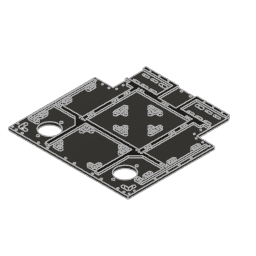
SumoBot-Chassis_5mm (Autodesk Fusion 360 design; units mm, degrees)
part number: 2026-04-02-11-57-34-569
Autodesk Fusion 360 part; units mm, degrees
(part 1 of 2)
sketch "Sketch1" plane through (0, 0, 0) normal (0, 0, 1) x (1, 0, 0)
  line L0 (67.5, 102.5) -> (-72.5, 102.5)
  line L1 (-102.5, 47.5) -> (-102.5, -97.5)
  line L2 (-102.5, -97.5) -> (97.5, -97.5)
  line L3 (97.5, -97.5) -> (97.5, 47.5)
  line L4 (-72.5, 102.5) -> (-72.5, 52.5)
  line L5 (67.5, 102.5) -> (67.5, 52.5)
  line L6 (-65.9, 77.5526) -> (-58.475, 77.6068)
  line L7 (-65.9, 74.3526) -> (-58.4517, 74.4069)
  line L8 (-51.9, 77.5526) -> (-44.1, 77.5526)
  line L9 (-51.9, 74.3526) -> (-44.1, 74.3526)
  arc A0 (-65.9, 77.5526) -> (-65.9, 74.3526) centre (-65.9, 75.9526) ccw
  arc A1 (-58.4517, 74.4069) -> (-58.475, 77.6068) centre (-58.4634, 76.0069) ccw
  arc A2 (-51.9, 77.5526) -> (-51.9, 74.3526) centre (-51.9, 75.9526) ccw
  arc A3 (-44.1, 74.3526) -> (-44.1, 77.5526) centre (-44.1, 75.9526) ccw
  arc A4 (-44.1, 90.4) -> (-44.1, 93.6) centre (-44.1, 92) ccw
  line L10 (-51.9, 90.4) -> (-44.1, 90.4)
  line L11 (-51.9, 93.6) -> (-44.1, 93.6)
  arc A5 (-51.9, 93.6) -> (-51.9, 90.4) centre (-51.9, 92) ccw
  line L12 (-65.9, 93.6) -> (-58.1, 93.6)
  arc A6 (-58.1, 90.4) -> (-58.1, 93.6) centre (-58.1, 92) ccw
  line L13 (-65.9, 90.4) -> (-58.1, 90.4)
  arc A7 (-65.9, 93.6) -> (-65.9, 90.4) centre (-65.9, 92) ccw
  line L14 (39.1, 74.3526) -> (46.9, 74.3526)
  arc A8 (39.1, 77.5526) -> (39.1, 74.3526) centre (39.1, 75.9526) ccw
  line L15 (39.1, 77.5526) -> (46.9, 77.5526)
  arc A9 (46.9, 74.3526) -> (46.9, 77.5526) centre (46.9, 75.9526) ccw
  arc A10 (53.1, 77.6) -> (53.1, 74.4) centre (53.1, 76) ccw
  line L16 (53.1, 74.4) -> (60.9, 74.4)
  line L17 (53.1, 77.6) -> (60.9, 77.6)
  arc A11 (60.9, 74.4) -> (60.9, 77.6) centre (60.9, 76) ccw
  arc A12 (39.1, 93.6474) -> (39.1, 90.4474) centre (39.1, 92.0474) ccw
  line L18 (39.1, 90.4474) -> (46.9, 90.4474)
  line L19 (39.1, 93.6474) -> (46.9, 93.6474)
  arc A13 (46.9, 90.4474) -> (46.9, 93.6474) centre (46.9, 92.0474) ccw
  line L20 (53.1, 90.3526) -> (60.9, 90.3526)
  arc A14 (53.1, 93.5526) -> (53.1, 90.3526) centre (53.1, 91.9526) ccw
  line L21 (53.1, 93.5526) -> (60.9, 93.5526)
  arc A15 (60.9, 90.3526) -> (60.9, 93.5526) centre (60.9, 91.9526) ccw
  arc A16 (-37.9, 77.6) -> (-37.9, 74.4) centre (-37.9, 76) ccw
  line L22 (-37.9, 77.6) -> (-30.1, 77.6)
  arc A17 (-30.1, 74.4) -> (-30.1, 77.6) centre (-30.1, 76) ccw
  line L23 (-37.9, 74.4) -> (-30.1, 74.4)
  line L24 (25.1, 77.5526) -> (32.9, 77.5526)
  arc A18 (32.9, 74.3526) -> (32.9, 77.5526) centre (32.9, 75.9526) ccw
  line L25 (25.1, 74.3526) -> (32.9, 74.3526)
  arc A19 (25.1, 77.5526) -> (25.1, 74.3526) centre (25.1, 75.9526) ccw
  line L26 (-72.5, 52.5) -> (-72.5, 47.5)
  line L27 (-72.5, 47.5) -> (-102.5, 47.5)
  line L28 (67.5, 52.5) -> (67.5, 47.5)
  line L29 (67.5, 47.5) -> (97.5, 47.5)
  line L30 (97.5, -97.5) -> (-102.5, -97.5)
  line L31 (-102.5, -97.5) -> (-102.5, -92.5)
  line L32 (97.5, -92.5) -> (97.5, -97.5)
  line L33 (75.5, -90.5) -> (45.5, -90.5)
  line L34 (45.5, -90.5) -> (45.5, -40.5)
  line L35 (45.5, -40.5) -> (75.5, -40.5)
  line L36 (75.5, -40.5) -> (75.5, -90.5)
  line L37 (-80.5, -90.5) -> (-50.5, -90.5)
  line L38 (-50.5, -90.5) -> (-50.5, -40.5)
  line L39 (-50.5, -40.5) -> (-80.5, -40.5)
  line L40 (-80.5, -40.5) -> (-80.5, -90.5)
  line L41 (79, -84.499) -> (85.4005, -84.4996)
  line L42 (78.9994, -89.499) -> (87.9249, -89.499)
  arc A20 (87.9249, -89.499) -> (90.3994, -86.6458) centre (87.9249, -86.9994) ccw
  arc A21 (79, -84.499) -> (78.9994, -89.499) centre (78.9994, -86.999) ccw
  line L43 (-93.4904, -89.5015) -> (-84.1058, -89.4532)
  line L44 (-90.5028, -84.4517) -> (-84.1181, -84.4532)
  arc A22 (-84.1058, -89.4532) -> (-84.1181, -84.4532) centre (-84.1187, -86.9532) ccw
  arc A23 (-95.5034, -86.5103) -> (-93.4904, -89.5015) centre (-93.0006, -86.999) ccw
  line L45 (90.3994, -86.9985) -> (90.3994, -78.099)
  arc A24 (87.8856, -89.499) -> (90.3994, -86.9985) centre (87.8994, -86.9991) ccw
  line L46 (85.4005, -84.4996) -> (85.3994, -78.0994)
  arc A25 (90.3994, -78.099) -> (85.3994, -78.0994) centre (87.8994, -78.099) ccw
  line L47 (-95.5009, -78.0957) -> (-95.5035, -86.9983)
  arc A26 (-90.5009, -78.0964) -> (-95.5009, -78.0957) centre (-93.0009, -78.0957) ccw
  line L48 (-90.5009, -78.0964) -> (-90.5028, -84.4517)
  arc A27 (-95.5035, -86.9983) -> (-92.9897, -89.499) centre (-93.0035, -86.999) ccw
  circle A28 centre (-65.5, -65.5) radius 15
  circle A29 centre (-65.5, -85) radius 2.1
  circle A30 centre (-65.5, -46) radius 2.1
  circle A31 centre (60.5, -85) radius 2.1
  circle A32 centre (60.5, -65.5) radius 15
  circle A33 centre (60.5, -46) radius 2.1
  line L49 (75.5, -80.5) -> (45.5, -80.5)
  line L50 (75.5, -50.5) -> (45.5, -50.5)
  line L51 (-50.5, -80.5) -> (-80.5, -80.5)
  line L52 (-50.5, -50.5) -> (-80.5, -50.5)
  line L53 (-70.5, 67.5) -> (-72.5, 67.5)
  line L54 (-70.5, 67.5) -> (-64.5, 67.5)
  line L55 (-64.5, 67.5) -> (-62.5, 67.5)
  circle A34 centre (-67.5, 48.623) radius 1.35
  circle A35 centre (-67.5, 48.623) radius 1.35
  circle A36 centre (-67.5, 59.5) radius 1.35
  line L56 (-64.5, 67.5) -> (-62.5, 67.5)
  line L57 (-70.5, 67.5) -> (-64.5, 67.5)
  line L58 (-70.5, 67.5) -> (-72.5, 67.5)
  circle A37 centre (62.5, 48.623) radius 1.35
  circle A38 centre (62.5, 59.5) radius 1.35
  line L59 (65.5, 67.5) -> (67.5, 67.5)
  line L60 (59.5, 67.5) -> (65.5, 67.5)
  line L61 (59.5, 67.5) -> (57.5, 67.5)
  circle A39 centre (-86.5, 43.5) radius 1.35
  circle A40 centre (-97.5, 43.5) radius 1.35
  circle A41 centre (-75.5, 43.5) radius 1.35
  circle A42 centre (92.5, 43.5) radius 1.35
  circle A43 centre (70.5, 43.5) radius 1.35
  circle A44 centre (81.5, 43.5) radius 1.35
  line L62 (-2.5, -97.5) -> (-2.5, 102.5)
  line L63 (-37, 94.5) -> (-29, 94.5)
  line L64 (-37, 89.5) -> (-29, 89.5)
  arc A45 (-37, 94.5) -> (-37, 89.5) centre (-37, 92) ccw
  arc A46 (-29, 89.5) -> (-29, 94.5) centre (-29, 92) ccw
  arc A47 (32, 89.5) -> (32, 94.5) centre (32, 92) ccw
  line L65 (24, 89.5) -> (32, 89.5)
  arc A48 (24, 94.5) -> (24, 89.5) centre (24, 92) ccw
  line L66 (24, 94.5) -> (32, 94.5)
  dimension "d64" = 200
  dimension "d104" = 6
  dimension "d107" = 2
  dimension "d110" = 6
  dimension "d111" = 2
  dimension "d165" = 50
  dimension "d166" = 10
  dimension "d167" = 30
  dimension "d247" = 2.7
  dimension "d248" = 2.7
  dimension "d249" = 2.7
  dimension "d250" = 2.7
  dimension "d251" = 2.7
  dimension "d252" = 2.7
  dimension "d253" = 2.7
  dimension "d254" = 2.7
  dimension "d256" = 2.7
  dimension "d257" = 2.7
  dimension "d258" = 4.2
  dimension "d259" = 4.2
  dimension "d260" = 4.2
  dimension "d261" = 4.2
  dimension "d263" = 1.6
  dimension "d264" = 2.5
  dimension "d265" = 2.5
  dimension "d266" = 2.5
  dimension "d268" = 2.5
  dimension "d269" = 2.5
  dimension "d270" = 2.5
  dimension "d271" = 2.5
  dimension "d272" = 2.5
  dimension "d273" = 2.5
  dimension "d274" = 2.5
  constraint horizontal L0
  constraint perpendicular L0 L1
  constraint parallel L0 L2
  constraint parallel L1 L3
  constraint vertical L4
  constraint vertical L5
  constraint tangent L6 A1
  constraint tangent L7 A1
  constraint tangent L8 A3
  constraint tangent L9 A3
  constraint tangent L12 A6
  constraint tangent A6 L13
  constraint tangent A4 L11
  constraint tangent A4 L10
  constraint tangent L15 A9
  constraint tangent L14 A9
  constraint tangent L17 A11
  constraint tangent L16 A11
  constraint tangent L19 A13
  constraint tangent L18 A13
  constraint tangent L21 A15
  constraint tangent L20 A15
  constraint tangent L22 A17
  constraint tangent A17 L23
  constraint tangent L24 A18
  constraint tangent A18 L25
  constraint perpendicular L1 L27
  constraint perpendicular L3 L29
  constraint horizontal L30
  constraint vertical L31
  constraint vertical L32
  constraint horizontal L33
  constraint vertical L34
  constraint horizontal L35
  constraint vertical L36
  constraint horizontal L37
  constraint vertical L38
  constraint horizontal L39
  constraint vertical L40
  constraint tangent L41 A20
  constraint tangent L42 A20
  constraint tangent L44 A22
  constraint tangent L43 A22
  constraint tangent L46 A25
  constraint tangent L45 A25
  constraint tangent L48 A27
  constraint tangent L47 A27
  constraint coincident L43 A27.end
  constraint coincident L47 A23.start
  constraint coincident L42 A24.start
  constraint coincident L45 A20.end
  constraint coincident L36 L49.start
  constraint perpendicular L34 L49
  constraint coincident L36 L50.start
  constraint coincident L34 L50.end
  constraint perpendicular L34 L50
  constraint coincident L4 L53.end
  constraint perpendicular L4 L53
  constraint parallel L54 L55
  constraint parallel L56 L57
  constraint midpoint L30 L62.start
  constraint midpoint L0 L62.end
  constraint perpendicular L0 L62
  constraint equal A6 A7
  constraint equal A4 A5
  constraint equal A5 A6
  constraint equal A0 A1
  constraint equal A0 A7
  constraint equal A2 A3
  constraint equal A2 A7
  constraint equal A16 A17
  constraint equal A7 A16
  constraint equal A12 A13
  constraint equal A14 A15
  constraint equal A10 A11
  constraint equal A8 A9
  constraint equal A18 A19
  constraint equal A7 A12
  constraint equal A7 A14
  constraint equal A7 A19
  constraint equal A7 A8
  constraint equal A7 A10
  constraint tangent L63 A46
  constraint parallel L0 L63
  constraint tangent L64 A46
  constraint parallel L63 L64
  constraint tangent A47 L66
  constraint tangent A47 L65
  constraint parallel L65 L66
  measures "d64" distance of L2.end L1.end
  measures "d104" distance of L53.start L54.end
  measures "d107" distance of L54.end L55.end
  measures "d110" distance of L53.start L54.end
  measures "d111" distance of L55.end L54.end
  measures "d165" distance of L37 L39
  measures "d166" distance of L39 L52
  measures "d167" distance of L38 L40
  measures "d247" diameter of A40
  measures "d248" diameter of A39
  measures "d249" diameter of A41
  measures "d250" diameter of A35
  measures "d251" diameter of A36
  measures "d252" diameter of A38
  measures "d253" diameter of A37
  measures "d254" diameter of A43
  measures "d256" diameter of A42
  measures "d257" diameter of A44
  measures "d258" diameter of A30
  measures "d259" diameter of A29
  measures "d260" diameter of A33
  measures "d261" diameter of A31
  measures "d263" radius of A7
  measures "d264" radius of A26
  measures "d265" radius of A22
  measures "d266" radius of A27
  measures "d268" radius of A25
  measures "d269" radius of A21
  measures "d270" radius of A24
  measures "d271" radius of A45
  measures "d272" radius of A46
  measures "d273" radius of A48
  measures "d274" radius of A47
extrude "Extrude1" add sketch "Sketch1" along normal blind 5 contours L0 L2 L3 L5 L28 L29 L30 L32 L62 | L0 L1 L2 L4 L26 L27 L30 L31 L62 | L33 L34 L36 L49 | L36 A32 L49 | L34 A32 L49 | L36 A32 L50 | L34 A32 L50 | L34 L35 L36 L50 | L37 L38 L40 L51 | L40 A28 L51 | L38 A28 L51 | L40 A28 L52 | L38 A28 L52 | L38 L39 L40 L52 makes body 1
fillet "Fillet1" radius 3 1 edges at (-2.5, 102.5, 0) on bodies 1
sketch "Sketch2" plane through (0, 0, 5) normal (0, 0, 1) x (-1, 0, 0)
  line L0 (-67.5, -102.5) -> (72.5, -102.5)
  line L1 (72.5, -102.5) -> (72.5, -47.5)
  line L2 (102.5, -47.5) -> (102.5, 97.5)
  line L3 (102.5, 97.5) -> (-97.5, 97.5)
  line L4 (-97.5, 97.5) -> (-97.5, -47.5)
  line L5 (-67.5, -47.5) -> (-67.5, -102.5)
  line L6 (72.5, -102.5) -> (22.5, -102.5)
  line L7 (22.5, -102.5) -> (22.5, -97.5)
  line L8 (22.5, -97.5) -> (72.5, -97.5)
  line L9 (72.5, -97.5) -> (72.5, -102.5)
  line L10 (27.5, -67.5) -> (72.5, -67.5)
  line L11 (72.5, -67.5) -> (72.5, -70.5)
  line L12 (-22.5, -67.5) -> (-67.5, -67.5)
  line L13 (-67.5, -67.5) -> (-67.5, -70.5)
  arc A0 (65.9, -77.5526) -> (65.9, -74.3526) centre (65.9, -75.9526) ccw
  line L14 (65.9, -77.5526) -> (58.475, -77.6068)
  arc A1 (58.4517, -74.4069) -> (58.475, -77.6068) centre (58.4634, -76.0069) ccw
  line L15 (58.4517, -74.4069) -> (65.9, -74.3526)
  arc A2 (-53.1, -93.5526) -> (-53.1, -90.3526) centre (-53.1, -91.9526) ccw
  line L16 (-53.1, -93.5526) -> (-60.9, -93.5526)
  arc A3 (-60.9, -90.3526) -> (-60.9, -93.5526) centre (-60.9, -91.9526) ccw
  line L17 (-60.9, -90.3526) -> (-53.1, -90.3526)
  arc A4 (65.9, -93.6) -> (65.9, -90.4) centre (65.9, -92) ccw
  line L18 (65.9, -93.6) -> (58.1, -93.6)
  arc A5 (58.1, -90.4) -> (58.1, -93.6) centre (58.1, -92) ccw
  line L19 (58.1, -90.4) -> (65.9, -90.4)
  arc A6 (-39.1, -77.5526) -> (-39.1, -74.3526) centre (-39.1, -75.9526) ccw
  line L20 (-39.1, -77.5526) -> (-46.9, -77.5526)
  arc A7 (-46.9, -74.3526) -> (-46.9, -77.5526) centre (-46.9, -75.9526) ccw
  line L21 (-46.9, -74.3526) -> (-39.1, -74.3526)
  arc A8 (-53.1, -77.6) -> (-53.1, -74.4) centre (-53.1, -76) ccw
  line L22 (-53.1, -77.6) -> (-60.9, -77.6)
  arc A9 (-60.9, -74.4) -> (-60.9, -77.6) centre (-60.9, -76) ccw
  line L23 (-60.9, -74.4) -> (-53.1, -74.4)
  arc A10 (51.9, -93.6) -> (51.9, -90.4) centre (51.9, -92) ccw
  line L24 (51.9, -93.6) -> (44.1, -93.6)
  arc A11 (44.1, -90.4) -> (44.1, -93.6) centre (44.1, -92) ccw
  line L25 (44.1, -90.4) -> (51.9, -90.4)
  arc A12 (51.9, -77.5526) -> (51.9, -74.3526) centre (51.9, -75.9526) ccw
  line L26 (51.9, -77.5526) -> (44.1, -77.5526)
  arc A13 (44.1, -74.3526) -> (44.1, -77.5526) centre (44.1, -75.9526) ccw
  line L27 (44.1, -74.3526) -> (51.9, -74.3526)
  arc A14 (-39.1, -93.6474) -> (-39.1, -90.4474) centre (-39.1, -92.0474) ccw
  line L28 (-39.1, -93.6474) -> (-46.9, -93.6474)
  arc A15 (-46.9, -90.4474) -> (-46.9, -93.6474) centre (-46.9, -92.0474) ccw
  line L29 (-46.9, -90.4474) -> (-39.1, -90.4474)
  arc A16 (-25.1, -77.5526) -> (-25.1, -74.3526) centre (-25.1, -75.9526) ccw
  line L30 (-25.1, -77.5526) -> (-32.9, -77.5526)
  arc A17 (-32.9, -74.3526) -> (-32.9, -77.5526) centre (-32.9, -75.9526) ccw
  line L31 (-32.9, -74.3526) -> (-25.1, -74.3526)
  arc A18 (37.9, -77.6) -> (37.9, -74.4) centre (37.9, -76) ccw
  line L32 (37.9, -77.6) -> (30.1, -77.6)
  arc A19 (30.1, -74.4) -> (30.1, -77.6) centre (30.1, -76) ccw
  line L33 (30.1, -74.4) -> (37.9, -74.4)
  line L34 (-67.5, -102.5) -> (-17.5, -102.5)
  line L35 (-17.5, -102.5) -> (-17.5, -97.5)
  line L36 (-17.5, -97.5) -> (-67.5, -97.5)
  line L37 (-67.5, -97.5) -> (-67.5, -102.5)
  line L38 (72.5, -47.5) -> (102.5, -47.5)
  line L39 (-97.5, -47.5) -> (-67.5, -47.5)
  circle A20 centre (65.5, 85) radius 2.1
  circle A21 centre (-60.5, 46) radius 2.1
  circle A22 centre (-60.5, 65.5) radius 15
  arc A23 (-79, 84.499) -> (-78.9994, 89.499) centre (-78.9994, 86.999) ccw
  line L40 (-79, 84.499) -> (-85.4005, 84.4996)
  line L41 (-85.4005, 84.4996) -> (-85.3994, 78.0994)
  arc A24 (-90.3994, 78.099) -> (-85.3994, 78.0994) centre (-87.8994, 78.099) ccw
  line L42 (-90.3994, 78.099) -> (-90.3994, 86.6458)
  arc A25 (-87.9249, 89.499) -> (-90.3994, 86.6458) centre (-87.9249, 86.9994) ccw
  arc A26 (-87.8856, 89.499) -> (-87.9132, 89.499) centre (-87.8994, 86.9991) ccw
  line L43 (-87.9249, 89.499) -> (-87.9132, 89.499)
  circle A27 centre (-60.5, 85) radius 2.1
  circle A28 centre (65.5, 46) radius 2.1
  circle A29 centre (65.5, 65.5) radius 15
  arc A30 (90.5009, 78.0964) -> (95.5009, 78.0957) centre (93.0009, 78.0957) ccw
  line L44 (90.5009, 78.0964) -> (90.5028, 84.4517)
  line L45 (90.5028, 84.4517) -> (84.1181, 84.4532)
  arc A31 (84.1058, 89.4532) -> (84.1181, 84.4532) centre (84.1187, 86.9532) ccw
  line L46 (84.1058, 89.4532) -> (93.4904, 89.5015)
  arc A32 (95.5034, 86.5103) -> (93.4904, 89.5015) centre (93.0006, 86.999) ccw
  line L47 (95.5034, 86.5103) -> (95.5009, 78.0957)
  circle A33 centre (67.5, -59.5) radius 1.35
  circle A34 centre (67.5, -48.623) radius 1.35
  circle A35 centre (-62.5, -48.623) radius 1.35
  circle A36 centre (-62.5, -59.5) radius 1.35
  circle A37 centre (75.5, -43.5) radius 1.35
  circle A38 centre (97.5, -43.5) radius 1.35
  circle A39 centre (86.5, -43.5) radius 1.35
  circle A40 centre (-81.5, -43.5) radius 1.35
  circle A41 centre (-92.5, -43.5) radius 1.35
  circle A42 centre (-70.5, -43.5) radius 1.35
  line L48 (72.5, -67.5) -> (64.5, -67.5)
  line L49 (64.5, -67.5) -> (64.5, -40.6151)
  line L50 (64.5, -40.6151) -> (102.5, -40.6151)
  line L51 (-67.5, -67.5) -> (-59.5, -67.5)
  line L52 (-59.5, -67.5) -> (-59.5, -40.6151)
  line L53 (-59.5, -40.6151) -> (-97.5, -40.6151)
  arc A43 (87.0072, -31.7917) -> (93, -32) centre (90, -32) ccw
  arc A44 (87.0072, -31.7917) -> (93, -32) centre (90, -32) ccw
  arc A45 (93, -24) -> (87, -24.0028) centre (90, -24) ccw
  line L54 (93, -32) -> (93, -24)
  line L55 (87.0072, -31.7917) -> (87, -24.0028)
  circle A46 centre (89.9963, -28) radius 1.425
  line L56 (87.0106, 8.0515) -> (87, 15.996)
  line L57 (93, 8) -> (93, 16)
  arc A47 (87.0104, 8.2491) -> (93, 8) centre (90, 8) ccw
  arc A48 (87.0104, 8.2491) -> (93, 8) centre (90, 8) ccw
  arc A49 (93, 16) -> (87, 15.996) centre (90, 16) ccw
  line L58 (87.0072, -31.7917) -> (87, -24.0028)
  arc A50 (87.0072, -31.7917) -> (93, -32) centre (90, -32) ccw
  line L59 (93, -32) -> (93, -24)
  arc A51 (93, -24) -> (87, -24.0028) centre (90, -24) ccw
  arc A52 (87.0104, 8.2491) -> (93, 8) centre (90, 8) ccw
  line L60 (93, 8) -> (93, 16)
  circle A53 centre (90, 8) radius 1.175
  arc A54 (93, 16) -> (87, 15.996) centre (90, 16) ccw
  line L61 (87.0106, 8.0515) -> (87, 15.996)
  line L62 (47.0072, -31.7917) -> (47, -24.0028)
  arc A55 (47.0072, -31.7917) -> (53, -32) centre (50, -32) ccw
  line L63 (53, -32) -> (53, -24)
  arc A56 (53, -24) -> (47, -24.0028) centre (50, -24) ccw
  circle A57 centre (50, -24) radius 1.175
  circle A58 centre (49.9963, -28) radius 1.425
  circle A59 centre (50, -32) radius 1.175
  line L64 (47.0106, 8.0515) -> (47, 15.996)
  arc A60 (47.0104, 8.2491) -> (53, 8) centre (50, 8) ccw
  line L65 (53, 8) -> (53, 16)
  arc A61 (53, 16) -> (47, 15.996) centre (50, 16) ccw
  circle A62 centre (50, 8) radius 1.175
  circle A63 centre (50, 12) radius 1.425
  circle A64 centre (50, 16) radius 1.175
  line L66 (-87.9928, -31.7917) -> (-88, -24.0028)
  arc A65 (-87.9928, -31.7917) -> (-82, -32) centre (-85, -32) ccw
  line L67 (-82, -32) -> (-82, -24)
  arc A66 (-82, -24) -> (-88, -24.0028) centre (-85, -24) ccw
  circle A67 centre (-85, -24) radius 1.175
  circle A68 centre (-85.0037, -28) radius 1.425
  circle A69 centre (-85, -32) radius 1.175
  line L68 (-87.9894, 8.0515) -> (-88, 15.996)
  arc A70 (-87.9896, 8.2491) -> (-82, 8) centre (-85, 8) ccw
  line L69 (-82, 8) -> (-82, 16)
  arc A71 (-82, 16) -> (-88, 15.996) centre (-85, 16) ccw
  circle A72 centre (-85, 8) radius 1.175
  circle A73 centre (-85, 12) radius 1.425
  circle A74 centre (-85, 16) radius 1.175
  arc A75 (-47.9928, -31.7917) -> (-42, -32) centre (-45, -32) ccw
  circle A76 centre (-45, -32) radius 1.175
  line L70 (-42, -32) -> (-42, -24)
  line L71 (-47.9928, -31.7917) -> (-48, -24.0028)
  circle A77 centre (-45.0037, -28) radius 1.425
  circle A78 centre (-45, -24) radius 1.175
  arc A79 (-42, -24) -> (-48, -24.0028) centre (-45, -24) ccw
  arc A80 (-47.9896, 8.2491) -> (-42, 8) centre (-45, 8) ccw
  line L72 (-47.9894, 8.0515) -> (-48, 15.996)
  arc A81 (-42, 16) -> (-48, 15.996) centre (-45, 16) ccw
  line L73 (-42, 8) -> (-42, 16)
  circle A82 centre (-45, 12) radius 1.425
  circle A83 centre (-45, 16) radius 1.175
  circle A84 centre (-45, 8) radius 1.175
  line L74 (-35, -59) -> (40, -59)
  line L75 (40, -59) -> (40, 21)
  line L76 (40, 21) -> (-35, 21)
  line L77 (-35, 21) -> (-35, -59)
  line L78 (64, -67.5) -> (64, -61.5)
  line L79 (64, -61.5) -> (-59, -61.5)
  line L80 (-59, -61.5) -> (-59, -67.5)
  line L81 (27.5, -67.5) -> (-22.5, -67.5)
  line L82 (102.5, -40.6151) -> (97.5, -40.6151)
  line L83 (97.5, -40.6151) -> (97.5, 91.5)
  line L84 (102.5, 97.5) -> (102.5, -40.6151)
  line L85 (-97.5, -40.6151) -> (-92.5, -40.6151)
  line L86 (-92.5, -40.6151) -> (-92.5, 91.5)
  line L87 (-97.5, 97.5) -> (-97.5, -40.6151)
  line L88 (94.5, 29.5) -> (59, 29.5)
  line L89 (47, 23.5) -> (47, -61.5)
  line L90 (47, -61.5) -> (53, -61.5)
  line L91 (53, -61.5) -> (53, 23.5)
  line L92 (-89.5, 29.5) -> (-54, 29.5)
  line L93 (-42, 23.5) -> (-42, -61.5)
  line L94 (-42, -61.5) -> (-48, -61.5)
  line L95 (-48, -61.5) -> (-48, 23.5)
  line L96 (41, 29.5) -> (-36, 29.5)
  line L97 (94.5, 23.5) -> (53, 23.5)
  line L98 (47, 23.5) -> (-42, 23.5)
  line L99 (-48, 23.5) -> (-89.5, 23.5)
  line L100 (22.5, -102.5) -> (17.5, -102.5)
  line L101 (17.5, -102.5) -> (17.5, -67.5)
  line L102 (17.5, -67.5) -> (22.5, -67.5)
  line L103 (22.5, -67.5) -> (22.5, -102.5)
  line L104 (-17.5, -102.5) -> (-12.5, -102.5)
  line L105 (-12.5, -102.5) -> (-12.5, -67.5)
  line L106 (-12.5, -67.5) -> (-17.5, -67.5)
  line L107 (-17.5, -67.5) -> (-17.5, -102.5)
  line L108 (22.5, -70.5) -> (72.5, -70.5)
  line L109 (-17.5, -70.5) -> (-67.5, -70.5)
  line L110 (97.5, 91.5) -> (-92.5, 91.5)
  line L111 (47, 41.5) -> (47, 91.5)
  line L112 (41, 29.5) -> (41, 91.5)
  line L113 (50.5, 40.5) -> (80.5, 40.5)
  line L114 (80.5, 40.5) -> (80.5, 90.5)
  line L115 (80.5, 90.5) -> (50.5, 90.5)
  line L116 (50.5, 90.5) -> (50.5, 40.5)
  line L117 (50.5, 40.5) -> (80.5, 90.5) construction
  line L118 (80.5, 40.5) -> (50.5, 90.5) construction
  line L119 (59, 29.5) -> (47, 41.5)
  line L120 (59, 29.5) -> (75.9706, 29.5) construction
  line L121 (-42, 41.5) -> (-42, 91.5)
  line L122 (-36, 91.5) -> (-36, 29.5)
  line L123 (-54, 29.5) -> (-42, 41.5)
  line L124 (87.0072, -31.7917) -> (87, -24.0028)
  arc A85 (87.0072, -31.7917) -> (93, -32) centre (90, -32) ccw
  line L125 (93, -32) -> (93, -24)
  arc A86 (93, -24) -> (87, -24.0028) centre (90, -24) ccw
  line L126 (87.0106, 8.0515) -> (87, 15.996)
  arc A87 (87.0104, 8.2491) -> (93, 8) centre (90, 8) ccw
  line L127 (93, 8) -> (93, 16)
  arc A88 (93, 16) -> (87, 15.996) centre (90, 16) ccw
  circle A89 centre (90, 16) radius 1.175
  line L128 (87.0106, 48.0515) -> (87, 55.996)
  arc A90 (87.0104, 48.2491) -> (93, 48) centre (90, 48) ccw
  line L129 (93, 48) -> (93, 56)
  circle A91 centre (90, 52) radius 1.425
  arc A92 (93, 56) -> (87, 55.996) centre (90, 56) ccw
  circle A93 centre (90, 48) radius 1.175
  line L130 (-87.9894, 48.0515) -> (-88, 55.996)
  arc A94 (-87.9896, 48.2491) -> (-82, 48) centre (-85, 48) ccw
  line L131 (-82, 48) -> (-82, 56)
  circle A95 centre (-85, 52) radius 1.425
  arc A96 (-82, 56) -> (-88, 55.996) centre (-85, 56) ccw
  circle A97 centre (-85, 56) radius 1.15
  line L132 (87.0106, 8.0515) -> (87, 15.996)
  arc A98 (87.0104, 8.2491) -> (93, 8) centre (90, 8) ccw
  line L133 (93, 8) -> (93, 16)
  circle A99 centre (90, 12) radius 1.425
  arc A100 (93, 16) -> (87, 15.996) centre (90, 16) ccw
  line L134 (93.9776, 23.529) -> (86.0331, 23.5184)
  arc A101 (93.7799, 23.5288) -> (94.029, 29.5184) centre (94.029, 26.5184) ccw
  line L135 (94.029, 29.5184) -> (86.029, 29.5184)
  circle A102 centre (90.029, 26.5184) radius 1.425
  arc A103 (86.029, 29.5184) -> (86.0331, 23.5184) centre (86.029, 26.5184) ccw
  circle A104 centre (94.029, 26.5184) radius 1.175
  circle A105 centre (86.029, 26.5184) radius 1.175
  line L136 (87.0106, 8.0515) -> (87, 15.996)
  arc A106 (87.0104, 8.2491) -> (93, 8) centre (90, 8) ccw
  line L137 (93, 8) -> (93, 16)
  arc A107 (93, 16) -> (87, 15.996) centre (90, 16) ccw
  line L138 (86, 63.5) -> (94, 63.5)
  circle A108 centre (90, 66.5) radius 1.425
  arc A109 (94, 63.5) -> (93.996, 69.5) centre (94, 66.5) ccw
  arc A110 (86.2491, 69.4896) -> (86, 63.5) centre (86, 66.5) ccw
  line L139 (86.0515, 69.4894) -> (93.996, 69.5)
  circle A111 centre (86, 66.5) radius 1.175
  circle A112 centre (94, 66.5) radius 1.175
  line L140 (46, 23.5) -> (54, 23.5)
  circle A113 centre (50, 26.5) radius 1.425
  arc A114 (54, 23.5) -> (53.996, 29.5) centre (54, 26.5) ccw
  arc A115 (46.2491, 29.4896) -> (46, 23.5) centre (46, 26.5) ccw
  line L141 (46.0515, 29.4894) -> (53.996, 29.5)
  circle A116 centre (46, 26.5) radius 1.175
  circle A117 centre (54, 26.5) radius 1.175
  line L142 (-82, 48) -> (-82, 56)
  arc A118 (-87.9896, 48.2491) -> (-82, 48) centre (-85, 48) ccw
  line L143 (-87.9894, 48.0515) -> (-88, 55.996)
  arc A119 (-82, 56) -> (-88, 55.996) centre (-85, 56) ccw
  circle A120 centre (-85, 56) radius 1.15
  circle A121 centre (-85, 48) radius 1.175
  line L144 (-81, 29.5) -> (-89, 29.5)
  arc A122 (-81.2491, 23.5104) -> (-81, 29.5) centre (-81, 26.5) ccw
  line L145 (-81.0515, 23.5106) -> (-88.996, 23.5)
  arc A123 (-89, 29.5) -> (-88.996, 23.5) centre (-89, 26.5) ccw
  circle A124 centre (-89, 26.5) radius 1.175
  circle A125 centre (-85, 26.5) radius 1.425
  circle A126 centre (-81, 26.5) radius 1.175
  line L146 (-89, 63.5) -> (-81, 63.5)
  arc A127 (-88.7509, 69.4896) -> (-89, 63.5) centre (-89, 66.5) ccw
  line L147 (-88.9485, 69.4894) -> (-81.004, 69.5)
  arc A128 (-81, 63.5) -> (-81.004, 69.5) centre (-81, 66.5) ccw
  circle A129 centre (-81, 66.5) radius 1.175
  circle A130 centre (-85, 66.5) radius 1.425
  circle A131 centre (-89, 66.5) radius 1.175
  line L148 (-49, 23.5) -> (-41, 23.5)
  arc A132 (-48.7509, 29.4896) -> (-49, 23.5) centre (-49, 26.5) ccw
  line L149 (-48.9485, 29.4894) -> (-41.004, 29.5)
  arc A133 (-41, 23.5) -> (-41.004, 29.5) centre (-41, 26.5) ccw
  circle A134 centre (-41, 26.5) radius 1.175
  circle A135 centre (-45, 26.5) radius 1.425
  circle A136 centre (-49, 26.5) radius 1.175
  line L150 (-82, 48) -> (-82, 56)
  arc A137 (-87.9896, 48.2491) -> (-82, 48) centre (-85, 48) ccw
  line L151 (-87.9894, 48.0515) -> (-88, 55.996)
  arc A138 (-82, 56) -> (-88, 55.996) centre (-85, 56) ccw
  circle A139 centre (-85, 56) radius 1.15
  line L152 (-88.9485, 69.4894) -> (-92.5, 69.4894)
  line L153 (-89, 63.5) -> (-92.5, 63.5)
  line L154 (93.996, 69.5) -> (97.5, 69.5047)
  line L155 (94, 63.5) -> (97.5, 63.5)
  line L156 (-92.5, -40.1151) -> (-89.5, -40.1151)
  line L157 (-89.5, -40.1151) -> (-89.5, 23.542)
  line L158 (-89.5, 29.458) -> (-89.5, 63.5)
  line L159 (93.4529, -40.6151) -> (93.4529, -40.1151)
  line L160 (97.5, -40.1151) -> (94.5, -40.1151)
  line L161 (94.5, -40.1151) -> (94.5, 23.5556)
  line L162 (94.5, 29.4812) -> (94.5, 63.5)
  line L163 (38, 34) -> (38, 42)
  arc A140 (38, 42) -> (32, 41.996) centre (35, 42) ccw
  circle A141 centre (35, 42) radius 1.175
  circle A142 centre (35, 38) radius 1.425
  line L164 (87.0106, 48.0515) -> (87, 55.996)
  arc A143 (87.0104, 48.2491) -> (93, 48) centre (90, 48) ccw
  line L165 (93, 48) -> (93, 56)
  arc A144 (93, 56) -> (87, 55.996) centre (90, 56) ccw
  circle A145 centre (90, 56) radius 1.175
  line L166 (27, 31) -> (35, 31)
  arc A146 (27.2491, 36.9896) -> (27, 31) centre (27, 34) ccw
  circle A147 centre (27, 34) radius 1.175
  circle A148 centre (31, 34) radius 1.425
  circle A149 centre (35, 34) radius 1.175
  line L167 (32.0067, 36.996) -> (32, 41.996)
  line L168 (27.0515, 36.9894) -> (32.0067, 36.996)
  arc A150 (35, 31) -> (38, 34.0027) centre (35, 34) ccw
  arc A151 (35, 37) -> (34.996, 37) centre (35, 34) ccw
  line L169 (-33, 42) -> (-33, 34)
  arc A152 (-33, 34) -> (-29.9973, 31) centre (-30, 34) ccw
  line L170 (-30, 31) -> (-22, 31)
  arc A153 (-22, 31) -> (-22.004, 37) centre (-22, 34) ccw
  line L171 (-27.004, 36.9933) -> (-22.004, 37)
  line L172 (-27.0106, 41.9485) -> (-27.004, 36.9933)
  arc A154 (-27.0104, 41.7509) -> (-33, 42) centre (-30, 42) ccw
  circle A155 centre (-30, 42) radius 1.175
  circle A156 centre (-30, 38) radius 1.425
  circle A157 centre (-30, 34) radius 1.175
  circle A158 centre (-26, 34) radius 1.425
  circle A159 centre (-22, 34) radius 1.175
  line L173 (38, 78) -> (38, 86)
  arc A160 (38, 86) -> (34.9973, 89) centre (35, 86) ccw
  line L174 (35, 89) -> (27, 89)
  arc A161 (27, 89) -> (27.004, 83) centre (27, 86) ccw
  line L175 (32.004, 83.0067) -> (27.004, 83)
  line L176 (32.0106, 78.0515) -> (32.004, 83.0067)
  arc A162 (32.0104, 78.2491) -> (38, 78) centre (35, 78) ccw
  circle A163 centre (35, 78) radius 1.175
  circle A164 centre (35, 82) radius 1.425
  circle A165 centre (35, 86) radius 1.175
  circle A166 centre (31, 86) radius 1.425
  circle A167 centre (27, 86) radius 1.175
  line L177 (-22, 89) -> (-30, 89)
  arc A168 (-30, 89) -> (-33, 85.9973) centre (-30, 86) ccw
  line L178 (-33, 86) -> (-33, 78)
  arc A169 (-33, 78) -> (-27, 78.004) centre (-30, 78) ccw
  line L179 (-27.0067, 83.004) -> (-27, 78.004)
  line L180 (-22.0515, 83.0106) -> (-27.0067, 83.004)
  arc A170 (-22.2491, 83.0104) -> (-22, 89) centre (-22, 86) ccw
  circle A171 centre (-22, 86) radius 1.175
  circle A172 centre (-26, 86) radius 1.425
  circle A173 centre (-30, 86) radius 1.175
  circle A174 centre (-30, 82) radius 1.425
  circle A175 centre (-30, 78) radius 1.175
  line L181 (-19.0017, 34.1) -> (24.0017, 34.1)
  line L182 (-30, 75) -> (-30, 45)
  line L183 (24.0017, 85.9) -> (-19.0017, 85.9)
  line L184 (35, 45) -> (35, 75)
  circle A176 centre (100, 29.4184) radius 1.35
  circle A177 centre (100, 9.4184) radius 1.35
  circle A178 centre (100, 49.4184) radius 1.35
  circle A179 centre (100, -10.5816) radius 1.35
  circle A180 centre (-95, -10.5816) radius 1.35
  circle A181 centre (-95, 9.4184) radius 1.35
  circle A182 centre (-95, 29.4184) radius 1.35
  circle A183 centre (-95, 49.4184) radius 1.35
  line L185 (-12.5, -96.5) -> (17.5, -96.5)
  circle A184 centre (-5, -99.5) radius 1.6
  circle A185 centre (10, -99.5) radius 1.6
  circle A186 centre (-5, 94.5) radius 1.6
  circle A187 centre (10, 94.5) radius 1.6
  circle A188 centre (-87.5, 94.5) radius 1.6
  circle A189 centre (92.5, 94.5) radius 1.6
  circle A190 centre (82.5, 94.5) radius 1.6
  circle A191 centre (-77.5, 94.5) radius 1.6
  circle A192 centre (-95, 84) radius 1.35
  circle A193 centre (-95, 93) radius 1.35
  circle A194 centre (100, 93) radius 1.35
  circle A195 centre (100, 84) radius 1.35
  arc A196 (-87.9928, -31.7917) -> (-82, -32) centre (-85, -32) ccw
  line L186 (-82, -32) -> (-82, -24)
  arc A197 (-82, -24) -> (-88, -24.0028) centre (-85, -24) ccw
  line L187 (-87.9928, -31.7917) -> (-88, -24.0028)
  line L188 (5.5, -45) -> (5.5, -40)
  arc A198 (5.5, -40) -> (-0.5, -40.004) centre (2.5, -40) ccw
  arc A199 (-5.5, -45) -> (-5.496, -51) centre (-5.5, -48) ccw
  line L189 (-0.4933, -45) -> (-5.5, -45)
  line L190 (-0.4933, -45) -> (-0.5, -40.004)
  arc A200 (10.2509, -50.9896) -> (10.5, -45) centre (10.5, -48) ccw
  circle A201 centre (10.5, -48) radius 1.175
  circle A202 centre (6.5, -48) radius 1.425
  line L191 (10.5, -45) -> (5.5, -45)
  line L192 (10.2509, -50.9896) -> (-5.496, -51)
  line L193 (10.2509, -50.9896) -> (-5.496, -51)
  arc A203 (10.2509, -50.9896) -> (10.5, -45) centre (10.5, -48) ccw
  line L194 (10.5, -45) -> (5.5, -45)
  line L195 (5.5, -45) -> (5.5, -40)
  arc A204 (5.5, -40) -> (-0.5, -40.004) centre (2.5, -40) ccw
  line L196 (-0.4933, -45) -> (-0.5, -40.004)
  arc A205 (-5.5, -45) -> (-5.496, -51) centre (-5.5, -48) ccw
  line L197 (-0.4933, -45) -> (-5.5, -45)
  circle A206 centre (2.5, -48) radius 1.175
  circle A207 centre (-1.5, -48) radius 1.425
  circle A208 centre (-5.5, -48) radius 1.175
  circle A209 centre (2.5, -44) radius 1.425
  circle A210 centre (2.5, -40) radius 1.175
  arc A211 (-29.4896, -26.7509) -> (-23.5, -27) centre (-26.5, -27) ccw
  line L198 (-23.5, -27) -> (-23.5, -22)
  line L199 (-23.5, -22) -> (-18.5, -22)
  arc A212 (-18.5, -22) -> (-18.504, -16) centre (-18.5, -19) ccw
  line L200 (-23.5, -16.0067) -> (-18.504, -16)
  line L201 (-23.5, -16.0067) -> (-23.5, -11)
  arc A213 (-23.5, -11) -> (-29.5, -11.004) centre (-26.5, -11) ccw
  line L202 (-29.4896, -26.7509) -> (-29.5, -11.004)
  circle A214 centre (-26.5, -27) radius 1.175
  circle A215 centre (-26.5, -23) radius 1.425
  circle A216 centre (-26.5, -19) radius 1.175
  circle A217 centre (-26.5, -15) radius 1.425
  circle A218 centre (-26.5, -11) radius 1.175
  circle A219 centre (-22.5, -19) radius 1.425
  circle A220 centre (-18.5, -19) radius 1.175
  arc A221 (-5.2509, 12.9896) -> (-5.5, 7) centre (-5.5, 10) ccw
  line L203 (-5.5, 7) -> (-0.5, 7)
  line L204 (-0.5, 7) -> (-0.5, 2)
  arc A222 (-0.5, 2) -> (5.5, 2.004) centre (2.5, 2) ccw
  line L205 (5.4933, 7) -> (5.5, 2.004)
  line L206 (5.4933, 7) -> (10.5, 7)
  arc A223 (10.5, 7) -> (10.496, 13) centre (10.5, 10) ccw
  line L207 (-5.2509, 12.9896) -> (10.496, 13)
  circle A224 centre (-5.5, 10) radius 1.175
  circle A225 centre (-1.5, 10) radius 1.425
  circle A226 centre (2.5, 10) radius 1.175
  circle A227 centre (6.5, 10) radius 1.425
  circle A228 centre (10.5, 10) radius 1.175
  circle A229 centre (2.5, 6) radius 1.425
  circle A230 centre (2.5, 2) radius 1.175
  arc A231 (34.4896, -11.2491) -> (28.5, -11) centre (31.5, -11) ccw
  line L208 (28.5, -11) -> (28.5, -16)
  line L209 (28.5, -16) -> (23.5, -16)
  arc A232 (23.5, -16) -> (23.504, -22) centre (23.5, -19) ccw
  line L210 (28.5, -21.9933) -> (23.504, -22)
  line L211 (28.5, -21.9933) -> (28.5, -27)
  arc A233 (28.5, -27) -> (34.5, -26.996) centre (31.5, -27) ccw
  line L212 (34.4896, -11.2491) -> (34.5, -26.996)
  circle A234 centre (31.5, -11) radius 1.175
  circle A235 centre (31.5, -15) radius 1.425
  circle A236 centre (31.5, -19) radius 1.175
  circle A237 centre (31.5, -23) radius 1.425
  circle A238 centre (31.5, -27) radius 1.175
  circle A239 centre (27.5, -19) radius 1.425
  circle A240 centre (23.5, -19) radius 1.175
  line L213 (2.498, -37) -> (2.502, -1)
  line L214 (-15.5, -18.998) -> (20.5, -19.002)
  line L215 (-8.5, -48.002) -> (-26.5, -48)
  line L216 (-26.502, -8) -> (-26.502, 10)
  line L217 (13.5, 10.002) -> (31.5, 9.9999)
  line L218 (31.502, -30) -> (31.5, -48)
  circle A241 centre (-57.5, -100) radius 1.175
  circle A242 centre (-42.5, -100) radius 1.175
  circle A243 centre (-27.5, -100) radius 1.175
  circle A244 centre (32.5, -100) radius 1.175
  circle A245 centre (47.5, -100) radius 1.175
  circle A246 centre (62.5, -100) radius 1.175
  circle A247 centre (40, 94.5) radius 1.6
  circle A248 centre (55, 94.5) radius 1.6
  circle A249 centre (-35, 94.5) radius 1.6
  circle A250 centre (-50, 94.5) radius 1.6
  line L219 (47.0106, -51.9485) -> (47, -44.004)
  arc A251 (53, -44) -> (47, -44.004) centre (50, -44) ccw
  line L220 (53, -52) -> (53, -44)
  arc A252 (47.0104, -51.7509) -> (53, -52) centre (50, -52) ccw
  circle A253 centre (50, -52) radius 1.175
  circle A254 centre (50, -48) radius 1.425
  circle A255 centre (50, -44) radius 1.175
  line L221 (-47.9894, -51.9485) -> (-48, -44.004)
  arc A256 (-42, -44) -> (-48, -44.004) centre (-45, -44) ccw
  line L222 (-42, -52) -> (-42, -44)
  arc A257 (-47.9896, -51.7509) -> (-42, -52) centre (-45, -52) ccw
  circle A258 centre (-45, -52) radius 1.175
  circle A259 centre (-45, -48) radius 1.425
  circle A260 centre (-45, -44) radius 1.175
  line L223 (-1.4485, -61.5106) -> (6.496, -61.5)
  arc A261 (6.5, -67.5) -> (6.496, -61.5) centre (6.5, -64.5) ccw
  line L224 (-1.5, -67.5) -> (6.5, -67.5)
  arc A262 (-1.2509, -61.5104) -> (-1.5, -67.5) centre (-1.5, -64.5) ccw
  circle A263 centre (-1.5, -64.5) radius 1.175
  circle A264 centre (2.5, -64.5) radius 1.425
  circle A265 centre (6.5, -64.5) radius 1.175
  line L225 (38.5515, -61.5106) -> (46.496, -61.5)
  arc A266 (46.5, -67.5) -> (46.496, -61.5) centre (46.5, -64.5) ccw
  arc A267 (38.7491, -61.5104) -> (38.5, -67.5) centre (38.5, -64.5) ccw
  line L226 (38.5, -67.5) -> (46.5, -67.5)
  circle A268 centre (42.5, -64.5) radius 1.425
  circle A269 centre (38.5, -64.5) radius 1.175
  circle A270 centre (46.5, -64.5) radius 1.175
  arc A271 (-33.5, -67.5) -> (-33.504, -61.5) centre (-33.5, -64.5) ccw
  line L227 (-41.5, -67.5) -> (-33.5, -67.5)
  arc A272 (-41.2509, -61.5104) -> (-41.5, -67.5) centre (-41.5, -64.5) ccw
  line L228 (-41.4485, -61.5106) -> (-33.504, -61.5)
  circle A273 centre (-33.5, -64.5) radius 1.175
  circle A274 centre (-37.5, -64.5) radius 1.425
  circle A275 centre (-41.5, -64.5) radius 1.175
  arc A276 (37, -94.5) -> (37, -89.5) centre (37, -92) ccw
  line L229 (37, -94.5) -> (29, -94.5)
  arc A277 (29, -89.5) -> (29, -94.5) centre (29, -92) ccw
  line L230 (29, -89.5) -> (37, -89.5)
  line L231 (-32, -89.5) -> (-24, -89.5)
  arc A278 (-24, -94.5) -> (-24, -89.5) centre (-24, -92) ccw
  line L232 (-24, -94.5) -> (-32, -94.5)
  arc A279 (-32, -89.5) -> (-32, -94.5) centre (-32, -92) ccw
  circle A280 centre (90, -32) radius 1.175
  circle A281 centre (90, -24) radius 1.175
  line L233 (-87.8856, 89.499) -> (-78.9994, 89.499)
  point P0 (65.5, 65.5)
  point P1 (90, 48)
  point P2 (-85, 48)
  point P3 (90, 8)
  point P4 (94.029, 26.5184)
  point P5 (90, 8)
  point P6 (35, 34)
  point P7 (90, 48)
  point P8 (-85.0037, -28)
  point P9 (2.5, 10)
  point P10 (2.5, -40)
  point P11 (2.5, -44)
  point P12 (-26.5, -19)
  dimension "d19" = 50
  dimension "d20" = 27
  dimension "d51" = 5
  dimension "d144" = 6
  dimension "d168" = 30
  dimension "d179" = 0.5
  dimension "d275" = 2.35
  dimension "d276" = 2.35
  dimension "d277" = 2.7
  dimension "d279" = 2.35
  dimension "d280" = 3.2
  dimension "d281" = 3.2
  dimension "d282" = 2.85
  dimension "d283" = 2.85
  constraint horizontal L6
  constraint vertical L7
  constraint horizontal L8
  constraint vertical L9
  constraint coincident L0.end L1.start
  constraint horizontal L10
  constraint vertical L11
  constraint coincident L1 L11.end
  constraint horizontal L12
  constraint vertical L13
  constraint coincident L5 L13.end
  constraint horizontal L34
  constraint vertical L35
  constraint horizontal L36
  constraint vertical L37
  constraint coincident L0.start L5.end
  constraint perpendicular L11 L48
  constraint perpendicular L48 L49
  constraint coincident L2 L50.end
  constraint perpendicular L2 L50
  constraint perpendicular L13 L51
  constraint perpendicular L12 L52
  constraint coincident L4 L53.end
  constraint perpendicular L4 L53
  constraint tangent A45 L54
  constraint coincident A43 A44.start
  constraint coincident A45 L55.end
  constraint tangent A45 L55
  constraint coincident L55 A43.start
  constraint coincident L55 A45.end
  constraint coincident L56.end A49
  constraint tangent L56 A49
  constraint tangent L57 A49
  constraint coincident L56 A47.start
  constraint coincident L56 A49.end
  constraint tangent L59 A51
  constraint coincident A43.start A50
  constraint coincident A45.end A51
  constraint tangent L58 A51
  constraint coincident A43.start L58
  constraint coincident A45.end L58
  constraint coincident L56.end A54
  constraint tangent A54 L61
  constraint tangent L60 A54
  constraint coincident A47.start L61
  constraint coincident L56.end L61
  constraint concentric A60 A62
  constraint concentric A56 A57
  constraint tangent L63 A56
  constraint concentric A61 A64
  constraint coincident L64.end A61
  constraint tangent L64 A61
  constraint tangent L65 A61
  constraint coincident A61.end L64
  constraint concentric A70 A72
  constraint concentric A66 A67
  constraint tangent L67 A66
  constraint concentric A71 A74
  constraint coincident L68.end A71
  constraint tangent L68 A71
  constraint tangent L69 A71
  constraint coincident A71.end L68
  constraint concentric A80 A84
  constraint concentric A78 A79
  constraint tangent L70 A79
  constraint concentric A81 A83
  constraint coincident L72.end A81
  constraint tangent L72 A81
  constraint tangent A81 L73
  constraint coincident A81.end L72
  constraint horizontal L74
  constraint perpendicular L74 L75
  constraint parallel L74 L76
  constraint parallel L75 L77
  constraint coincident L10 L78.start
  constraint perpendicular L52 L79
  constraint coincident L12 L80.end
  constraint perpendicular L12 L80
  constraint horizontal L82
  constraint vertical L83
  constraint vertical L84
  constraint horizontal L85
  constraint vertical L86
  constraint vertical L87
  constraint perpendicular L86 L97
  constraint perpendicular L83 L88
  constraint vertical L89
  constraint horizontal L90
  constraint vertical L91
  constraint perpendicular L86 L92
  constraint vertical L93
  constraint horizontal L94
  constraint vertical L95
  constraint perpendicular L93 L96
  constraint collinear L97 L98
  constraint collinear L98 L99
  constraint horizontal L100
  constraint vertical L101
  constraint horizontal L102
  constraint vertical L103
  constraint coincident L81 L101.end
  constraint horizontal L104
  constraint vertical L105
  constraint horizontal L106
  constraint vertical L107
  constraint coincident L81 L105.end
  constraint coincident L103 L108.start
  constraint perpendicular L11 L108
  constraint coincident L107 L109.start
  constraint perpendicular L13 L109
  constraint perpendicular L86 L110
  constraint coincident L110 L111.end
  constraint perpendicular L110 L111
  constraint coincident L110 L112.end
  constraint perpendicular L110 L112
  constraint horizontal L113
  constraint perpendicular L113 L114
  constraint parallel L113 L115
  constraint parallel L114 L116
  constraint coincident L117 P0
  constraint coincident L118 P0
  constraint coincident P0 A29.centre
  constraint horizontal L120
  constraint coincident L110 L121.end
  constraint perpendicular L110 L121
  constraint coincident L110 L122.start
  constraint perpendicular L96 L122
  constraint concentric A88 A89
  constraint coincident A43.start A85
  constraint coincident A43.start L124
  constraint coincident L56.end A88
  constraint tangent L126 A88
  constraint coincident L56.end L126
  constraint coincident L128.end A92
  constraint tangent L128 A92
  constraint coincident A90.start L128
  constraint coincident A92.end L128
  constraint coincident L130.end A96
  constraint tangent L130 A96
  constraint coincident A94.start L130
  constraint coincident A96.end L130
  constraint coincident L56.end A100
  constraint tangent L132 A100
  constraint coincident A47.start L132
  constraint coincident L56.end L132
  constraint coincident L134.end A103
  constraint tangent L134 A103
  constraint coincident A101.start L134
  constraint coincident A103.end L134
  constraint coincident L56.end A107
  constraint tangent L136 A107
  constraint coincident A47.start L136
  constraint coincident L56.end L136
  constraint coincident L139.end A109
  constraint tangent A109 L139
  constraint coincident A110.start L139
  constraint coincident A109.end L139
  constraint coincident L141.end A114
  constraint tangent A114 L141
  constraint coincident A115.start L141
  constraint coincident A114.end L141
  constraint coincident L130.end A119
  constraint tangent L143 A119
  constraint coincident A94.start L143
  constraint coincident L130.end L143
  constraint coincident L145.end A123
  constraint tangent L145 A123
  constraint coincident A122.start L145
  constraint coincident A123.end L145
  constraint coincident L147.end A128
  constraint tangent L147 A128
  constraint coincident A127.start L147
  constraint coincident A128.end L147
  constraint coincident L149.end A133
  constraint tangent L149 A133
  constraint coincident A132.start L149
  constraint coincident A133.end L149
  constraint coincident L130.end A138
  constraint tangent L151 A138
  constraint coincident A94.start L151
  constraint coincident L130.end L151
  constraint coincident L86 L152.end
  constraint perpendicular L86 L152
  constraint coincident L86 L153.end
  constraint tangent A127 L153
  constraint coincident L83 L154.end
  constraint tangent A109 L154
  constraint coincident L83 L155.end
  constraint tangent A109 L155
  constraint coincident L86 L156.start
  constraint perpendicular L86 L156
  constraint coincident L153 L158.end
  constraint perpendicular L153 L157
  constraint coincident A123 L157.end
  constraint collinear L157 L158
  constraint coincident A123 L158.start
  constraint coincident L158 L92.start
  constraint coincident L157 L99.end
  constraint coincident L50 L159.start
  constraint perpendicular L50 L159
  constraint coincident L83 L160.start
  constraint perpendicular L83 L160
  constraint vertical L161
  constraint coincident L155 L162.end
  constraint coincident L97.start L161
  constraint coincident L88.start L161
  constraint coincident A101 L161.end
  constraint collinear L161 L162
  constraint coincident A101 L162.start
  constraint coincident L167.end A140
  constraint coincident L128.end A144
  constraint tangent L164 A144
  constraint coincident A90.start L164
  constraint coincident L128.end L164
  constraint tangent L168 A150
  constraint coincident A146.start L168
  constraint coincident A151.end L168
  constraint coincident A146 L181.end
  constraint coincident A151.start A150
  constraint coincident L163 A150.end
  constraint concentric A150 A151
  constraint coincident A140 L184.start
  constraint coincident L171.end A153
  constraint tangent A152 L172
  constraint coincident A154.start L172
  constraint coincident A152.end L170
  constraint coincident L175.end A161
  constraint tangent A160 L176
  constraint coincident A162.start L176
  constraint coincident A160.end L174
  constraint coincident L179.end A169
  constraint tangent A168 L180
  constraint coincident A170.start L180
  constraint coincident A168.end L178
  constraint coincident A153 L181.start
  constraint coincident A154 L182.end
  constraint coincident A169 L182.start
  constraint coincident A170 L183.end
  constraint coincident A161 L183.start
  constraint coincident A162 L184.end
  constraint coincident L105 L185.start
  constraint perpendicular L105 L185
  constraint tangent L186 A197
  constraint midpoint A198 L213.start
  constraint midpoint A222 L213.end
  constraint midpoint A212 L214.start
  constraint midpoint A232 L214.end
  constraint perpendicular L213 L214
  constraint midpoint A205 L215.start
  constraint parallel L214 L215
  constraint midpoint A213 L216.start
  constraint vertical L216
  constraint midpoint A223 L217.start
  constraint midpoint A233 L218.start
  constraint tangent A251 L220
  constraint tangent A256 L222
  constraint coincident L223.end A261
  constraint tangent L223 A261
  constraint coincident A262.start L223
  constraint coincident A261.end L223
  constraint coincident L225.end A266
  constraint tangent L225 A266
  constraint coincident A267.start L225
  constraint coincident A266.end L225
  constraint coincident L228.end A271
  constraint tangent A271 L228
  constraint coincident A272.start L228
  constraint coincident A271.end L228
  constraint equal A67 A69
  constraint equal A69 A258
  constraint equal A258 A260
  constraint equal A69 A76
  constraint equal A76 A78
  constraint equal A72 A74
  constraint equal A83 A84
  constraint equal A69 A72
  constraint equal A69 A84
  constraint equal A273 A275
  constraint equal A69 A275
  constraint equal A263 A265
  constraint equal A69 A263
  constraint equal A269 A270
  constraint equal A69 A269
  constraint equal A253 A255
  constraint equal A57 A59
  constraint equal A62 A64
  constraint equal A69 A253
  constraint equal A59 A69
  constraint equal A62 A69
  constraint equal A53 A89
  constraint equal A53 A69
  constraint concentric A43 A280
  constraint concentric A51 A281
  constraint equal A280 A281
  constraint equal A69 A280
  constraint equal A104 A105
  constraint equal A116 A117
  constraint equal A69 A105
  constraint equal A69 A116
  constraint equal A134 A136
  constraint equal A69 A136
  constraint equal A124 A126
  constraint equal A69 A124
  constraint equal A129 A131
  constraint equal A69 A129
  constraint equal A69 A121
  constraint equal A93 A145
  constraint equal A111 A112
  constraint equal A69 A111
  constraint equal A69 A93
  constraint equal A206 A208
  constraint equal A206 A210
  constraint equal A69 A206
  constraint equal A201 A206
  constraint equal A216 A218
  constraint equal A214 A216
  constraint equal A216 A220
  constraint equal A69 A216
  constraint equal A224 A226
  constraint equal A226 A228
  constraint equal A226 A230
  constraint equal A69 A226
  constraint equal A234 A236
  constraint equal A236 A240
  constraint equal A69 A236
  constraint equal A236 A238
  constraint equal A147 A149
  constraint equal A141 A149
  constraint equal A165 A167
  constraint equal A163 A165
  constraint equal A157 A159
  constraint equal A155 A157
  constraint equal A173 A175
  constraint equal A171 A173
  constraint equal A149 A173
  constraint equal A149 A165
  constraint equal A149 A157
  constraint equal A177 A179
  constraint equal A176 A179
  constraint equal A178 A179
  constraint equal A179 A195
  constraint equal A179 A194
  constraint equal A180 A181
  constraint equal A180 A182
  constraint equal A180 A183
  constraint equal A180 A192
  constraint equal A180 A193
  constraint equal A179 A180
  constraint equal A245 A246
  constraint equal A244 A246
  constraint equal A243 A246
  constraint equal A242 A246
  constraint equal A241 A246
  constraint equal A184 A185
  constraint equal A186 A187
  constraint equal A187 A249
  constraint equal A187 A250
  constraint equal A187 A191
  constraint equal A187 A188
  constraint equal A187 A247
  constraint equal A187 A248
  constraint equal A187 A190
  constraint equal A187 A189
  constraint equal A46 A268
  constraint equal A46 A254
  constraint equal A46 A58
  constraint equal A46 A99
  constraint equal A46 A63
  constraint equal A46 A237
  constraint equal A46 A239
  constraint equal A46 A235
  constraint equal A46 A264
  constraint equal A46 A274
  constraint equal A46 A259
  constraint equal A46 A202
  constraint equal A46 A207
  constraint equal A46 A209
  constraint equal A217 A219
  constraint equal A46 A219
  constraint equal A215 A219
  constraint equal A225 A229
  constraint equal A227 A229
  constraint equal A46 A229
  constraint equal A46 A82
  constraint equal A46 A77
  constraint equal A46 A68
  constraint equal A46 A73
  constraint equal A46 A125
  constraint equal A46 A135